Autodesk Inventor part; units mm, degrees
(part 2 of 2)
  spline S102 degree 2 poles (164.944, 6.0057) (164.944, 6.7577) (165.6831, 7.5907) (166.286, 7.5907) knots 0 0 0 1 2 2 2
  spline S103 degree 2 poles (166.286, 7.5907) (166.8954, 7.5907) (167.6247, 6.7609) (167.6247, 6.0057) knots 0 0 0 1 2 2 2
  spline S104 degree 2 poles (167.1028, 6.0057) (167.1028, 6.5891) (166.6782, 7.1564) (166.286, 7.1564) knots 0 0 0 1 2 2 2
  spline S105 degree 2 poles (166.286, 7.1564) (165.8938, 7.1564) (165.4659, 6.5891) (165.4659, 6.0057) knots 0 0 0 1 2 2 2
  spline S106 degree 2 poles (165.4659, 6.0057) (165.4659, 5.4384) (165.8938, 4.8549) (166.286, 4.8549) knots 0 0 0 1 2 2 2
  spline S107 degree 2 poles (166.286, 4.8549) (166.675, 4.8549) (167.1028, 5.4287) (167.1028, 6.0057) knots 0 0 0 1 2 2 2
  line L93 (170.4772, 4.5048) -> (169.9716, 4.5048)
  line L94 (169.9716, 4.5048) -> (169.9716, 4.8355)
  spline S108 degree 2 poles (169.9716, 4.8355) (169.7382, 4.6313) (169.32, 4.4206) (169.0607, 4.4206) knots 0 0 0 1 2 2 2
  spline S109 degree 2 poles (169.0607, 4.4206) (168.8662, 4.4206) (168.5194, 4.5502) (168.3929, 4.6896) knots 0 0 0 1 2 2 2
  spline S110 degree 2 poles (168.3929, 4.6896) (168.2633, 4.829) (168.1207, 5.2536) (168.1207, 5.5583) knots 0 0 0 1 2 2 2
  line L95 (168.1207, 5.5583) -> (168.1207, 7.5065)
  line L96 (168.1207, 7.5065) -> (168.6263, 7.5065)
  line L97 (168.6263, 7.5065) -> (168.6263, 5.795)
  spline S111 degree 2 poles (168.6263, 5.795) (168.6263, 5.5551) (168.662, 5.2407) (168.7236, 5.124) knots 0 0 0 1 2 2 2
  spline S112 degree 2 poles (168.7236, 5.124) (168.7852, 5.0073) (168.9959, 4.9003) (169.1936, 4.9003) knots 0 0 0 1 2 2 2
  spline S113 degree 2 poles (169.1936, 4.9003) (169.3784, 4.9003) (169.7965, 5.111) (169.9716, 5.2634) knots 0 0 0 1 2 2 2
  line L98 (169.9716, 5.2634) -> (169.9716, 7.5065)
  line L99 (169.9716, 7.5065) -> (170.4772, 7.5065)
  line L100 (170.4772, 7.5065) -> (170.4772, 4.5048)
  spline S114 degree 2 poles (174.5291, 4.4335) (174.1401, 4.4335) (173.4821, 4.6961) (173.2422, 4.9587) knots 0 0 0 1 2 2 2
  spline S115 degree 2 poles (173.2422, 4.9587) (173.0023, 5.218) (172.7398, 5.9959) (172.7398, 6.5016) knots 0 0 0 1 2 2 2
  spline S116 degree 2 poles (172.7398, 6.5016) (172.7398, 7.004) (172.9959, 7.7496) (173.239, 8.0251) knots 0 0 0 1 2 2 2
  spline S117 degree 2 poles (173.239, 8.0251) (173.4788, 8.2941) (174.1336, 8.5762) (174.5388, 8.5762) knots 0 0 0 1 2 2 2
  spline S118 degree 2 poles (174.5388, 8.5762) (174.7398, 8.5762) (175.0931, 8.5178) (175.2422, 8.4724) knots 0 0 0 1 2 2 2
  spline S119 degree 2 poles (175.2422, 8.4724) (175.3719, 8.4303) (175.6409, 8.3104) (175.7738, 8.239) knots 0 0 0 1 2 2 2
  line L101 (175.7738, 8.239) -> (175.7738, 7.5972)
  line L102 (175.7738, 7.5972) -> (175.7317, 7.5972)
  spline S120 degree 2 poles (175.7317, 7.5972) (175.6604, 7.6621) (175.44, 7.8436) (175.2811, 7.9311) knots 0 0 0 1 2 2 2
  spline S121 degree 2 poles (175.2811, 7.9311) (175.1288, 8.0154) (174.769, 8.1223) (174.5356, 8.1223) knots 0 0 0 1 2 2 2
  spline S122 degree 2 poles (174.5356, 8.1223) (174.2795, 8.1223) (173.8224, 7.9116) (173.6506, 7.7107) knots 0 0 0 1 2 2 2
  spline S123 degree 2 poles (173.6506, 7.7107) (173.4821, 7.5065) (173.2941, 6.8873) (173.2941, 6.5016) knots 0 0 0 1 2 2 2
  spline S124 degree 2 poles (173.2941, 6.5016) (173.2941, 6.0899) (173.4918, 5.4967) (173.6636, 5.2925) knots 0 0 0 1 2 2 2
  spline S125 degree 2 poles (173.6636, 5.2925) (173.8322, 5.0948) (174.2827, 4.8938) (174.5356, 4.8938) knots 0 0 0 1 2 2 2
  spline S126 degree 2 poles (174.5356, 4.8938) (174.7657, 4.8938) (175.1579, 5.0073) (175.3103, 5.0916) knots 0 0 0 1 2 2 2
  spline S127 degree 2 poles (175.3103, 5.0916) (175.4562, 5.1758) (175.6733, 5.3509) (175.7349, 5.4125) knots 0 0 0 1 2 2 2
  line L103 (175.7349, 5.4125) -> (175.7738, 5.4125)
  line L104 (175.7738, 5.4125) -> (175.7738, 4.7771)
  spline S128 degree 2 poles (175.7738, 4.7771) (175.6409, 4.7155) (175.4075, 4.6021) (175.2422, 4.5502) knots 0 0 0 1 2 2 2
  spline S129 degree 2 poles (175.2422, 4.5502) (175.0672, 4.4919) (174.769, 4.4335) (174.5291, 4.4335) knots 0 0 0 1 2 2 2
  point P0 (0, 0)
  constraints: 2 other
extrude "Extrusión8" cut sketch "Boceto10" against normal blind 0.3
sketch "Boceto11" plane through (0, 0, 0) normal (0, -1, 0) x (1, 0, 0)
  line L0 (10.005, -7.4262) -> (-19.8869, -7.4262) construction
  line L1 (-19.8869, -7.4262) -> (-19.8869, 2.4029) construction
  line L2 (-19.8869, 2.4029) -> (10.005, 2.4029) construction
  line L3 (10.005, 2.4029) -> (10.005, -7.4262) construction
  line L4 (7.6083, -4.8816) -> (7.9406, -4.8816)
  line L5 (7.9406, -4.8816) -> (7.9406, -7.0351)
  line L6 (7.9406, -7.0351) -> (8.5929, -5.5704)
  line L7 (8.5929, -5.5704) -> (8.7955, -5.5704)
  line L8 (8.7955, -5.5704) -> (9.4418, -7.0351)
  line L9 (9.4418, -7.0351) -> (9.4418, -4.8816)
  line L10 (9.4418, -4.8816) -> (9.7518, -4.8816)
  line L11 (9.7518, -4.8816) -> (9.7518, -7.3816)
  line L12 (9.7518, -7.3816) -> (9.298, -7.3816)
  line L13 (9.298, -7.3816) -> (8.674, -5.9898)
  line L14 (8.674, -5.9898) -> (8.0703, -7.3816)
  line L15 (8.0703, -7.3816) -> (7.6083, -7.3816)
  line L16 (7.6083, -7.3816) -> (7.6083, -4.8816)
  line L17 (6.5184, -4.8816) -> (6.5184, -7.0858)
  line L18 (6.5184, -7.0858) -> (7.3571, -7.0858)
  line L19 (7.3571, -7.0858) -> (7.3571, -7.3816)
  line L20 (7.3571, -7.3816) -> (5.3474, -7.3816)
  line L21 (5.3474, -7.3816) -> (5.3474, -7.0858)
  line L22 (5.3474, -7.0858) -> (6.1861, -7.0858)
  line L23 (6.1861, -7.0858) -> (6.1861, -4.8816)
  line L24 (6.1861, -4.8816) -> (6.5184, -4.8816)
  spline S0 degree 2 poles (4.1177, -4.837) (4.3608, -4.837) (4.772, -5.0011) (4.922, -5.1652) knots 0 0 0 1 2 2 2
  spline S1 degree 2 poles (4.922, -5.1652) (5.0719, -5.3273) (5.236, -5.8135) (5.236, -6.1296) knots 0 0 0 1 2 2 2
  spline S2 degree 2 poles (5.236, -6.1296) (5.236, -6.4436) (5.0759, -6.9095) (4.924, -7.0817) knots 0 0 0 1 2 2 2
  spline S3 degree 2 poles (4.924, -7.0817) (4.7741, -7.2499) (4.3648, -7.4262) (4.1116, -7.4262) knots 0 0 0 1 2 2 2
  spline S4 degree 2 poles (4.1116, -7.4262) (3.986, -7.4262) (3.7652, -7.3897) (3.672, -7.3613) knots 0 0 0 1 2 2 2
  spline S5 degree 2 poles (3.672, -7.3613) (3.5909, -7.335) (3.4228, -7.26) (3.3397, -7.2155) knots 0 0 0 1 2 2 2
  line L25 (3.3397, -7.2155) -> (3.3397, -6.8143)
  line L26 (3.3397, -6.8143) -> (3.366, -6.8143)
  spline S6 degree 2 poles (3.366, -6.8143) (3.4106, -6.8548) (3.5484, -6.9683) (3.6476, -7.023) knots 0 0 0 1 2 2 2
  spline S7 degree 2 poles (3.6476, -7.023) (3.7429, -7.0757) (3.9677, -7.1425) (4.1136, -7.1425) knots 0 0 0 1 2 2 2
  spline S8 degree 2 poles (4.1136, -7.1425) (4.2737, -7.1425) (4.5593, -7.0108) (4.6667, -6.8852) knots 0 0 0 1 2 2 2
  spline S9 degree 2 poles (4.6667, -6.8852) (4.772, -6.7576) (4.8895, -6.3706) (4.8895, -6.1296) knots 0 0 0 1 2 2 2
  spline S10 degree 2 poles (4.8895, -6.1296) (4.8895, -5.8723) (4.766, -5.5015) (4.6586, -5.3739) knots 0 0 0 1 2 2 2
  spline S11 degree 2 poles (4.6586, -5.3739) (4.5532, -5.2503) (4.2716, -5.1247) (4.1136, -5.1247) knots 0 0 0 1 2 2 2
  spline S12 degree 2 poles (4.1136, -5.1247) (3.9698, -5.1247) (3.7246, -5.1956) (3.6294, -5.2483) knots 0 0 0 1 2 2 2
  spline S13 degree 2 poles (3.6294, -5.2483) (3.5382, -5.3009) (3.4025, -5.4103) (3.364, -5.4488) knots 0 0 0 1 2 2 2
  line L27 (3.364, -5.4488) -> (3.3397, -5.4488)
  line L28 (3.3397, -5.4488) -> (3.3397, -5.0518)
  spline S14 degree 2 poles (3.3397, -5.0518) (3.4228, -5.0133) (3.5686, -4.9424) (3.672, -4.9099) knots 0 0 0 1 2 2 2
  spline S15 degree 2 poles (3.672, -4.9099) (3.7814, -4.8735) (3.9677, -4.837) (4.1177, -4.837) knots 0 0 0 1 2 2 2
  point P0 (0, 0)
  constraints: 2 other
extrude "Extrusión9" cut sketch "Boceto11" against normal blind 0.3
sketch "Boceto12" plane through (0, 2, 0) normal (0, 1, 0) x (1, 0, 0)
  line L0 (89.4618, 42) -> (98.4618, 42) projected
  line L1 (90, 53.25) -> (0, 53.25)
  line L2 (90, 53.25) -> (180, 53.25)
  line L3 (90, 51.75) -> (180, 51.75)
  line L4 (90, 51.75) -> (0, 51.75)
  line L5 (0, 53.25) -> (15, 53.25)
  line L6 (15, 53.25) -> (15, 51.75)
  line L7 (180, 53.25) -> (165, 53.25)
  line L8 (165, 53.25) -> (165, 51.75)
  dimension "d377" = 15
  constraints: 16 end point, 5 point on line, 2 perpendicular
  measures "d377" distance of L1.end L5.end
extrude "Extrusión10" cut sketch "Boceto12" against normal blind 0.4
